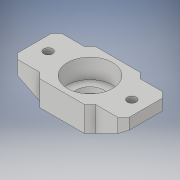
# Autodesk Inventor part: Sharrnir
Saved by Autodesk Inventor 2019.4 (Build 234330000, 330)
## iProperties
Created: 2019-04-09
Part Number: Sharrnir
Material: Типовые
Document SubType Name: Modeling
Designer: NoName
Density: 1 g/cm^3
Appearance: По умолчанию
Author: NoName
Autodesk Inventor part; units mm, degrees
ref_plane "YZ Plane" through (0, 0, 0) normal (1, 0, 0) x (0, 1, 0)
ref_plane "XZ Plane" through (0, 0, 0) normal (0, 1, 0) x (-1, 0, 0)
ref_plane "XY Plane" through (0, 0, 0) normal (0, 0, 1) x (1, 0, 0)
sketch "Эскиз1" plane through (0, 0, 0) normal (0, 1, 0) x (-1, 0, 0)
  circle A0 centre (0, 0) radius 5
  line L0 (8, 10) -> (-8, 10)
  line L1 (-10, 8) -> (-10, -8)
  line L2 (-8, -10) -> (8, -10)
  line L3 (10, -8) -> (10, 8)
  circle A1 centre (0, 0) radius 8 construction
  line L4 (8, 10) -> (10, 8)
  line L5 (10, -8) -> (8, -10)
  line L6 (-8, -10) -> (-10, -8)
  line L7 (-8, 10) -> (-10, 8)
  point P0 (10, 10)
  point P1 (-10, -10)
  point P2 (-10, 10)
  point P3 (10, -10)
  point P4 (0, -10)
  point P5 (10, 0)
  dimension "d0" = 10
  dimension "d3" = 16
  dimension "d4" = 20
  dimension "d5" = 20
  dimension "d6" = 2
  dimension "d7" = 2
  dimension "d8" = 2
  dimension "d9" = 2
  dimension "d10" = 2
  dimension "d11" = 2
  dimension "d12" = 2
  dimension "d13" = 2
  constraints: 16 end point, 8 point on line, 2 centre point, 2 coincident, 2 midpoint, 2 parallel, 1 horizontal, 1 horizontal alignment, 1 perpendicular, 1 vertical alignment
  measures "d0" diameter of A0
  measures "d3" diameter of A1
  measures "d4" distance between parallel lines of L2 L0
  measures "d5" distance between parallel lines of L3 L1
  measures "d6" distance of L0.start point (10, 10)
  measures "d7" distance of L3.end point (10, 10)
  measures "d8" distance of L3.start point (10, -10)
  measures "d9" distance of L2.end point (10, -10)
  measures "d10" distance of L2.start point (-10, -10)
  measures "d11" distance of L1.end point (-10, -10)
  measures "d12" distance of L0.end point (-10, 10)
  measures "d13" distance of L1.start point (-10, 10)
extrude "Выдавливание1" add sketch "Эскиз1" along normal blind 5
sketch "Эскиз4" plane through (0, 5, 0) normal (0, 1, 0) x (1, 0, 0)
  line L0 (12.8246, 0) -> (14.4123, 2.75) construction
  line L1 (14.4123, 2.75) -> (17.5877, 2.75) construction
  line L2 (17.5877, 2.75) -> (19.1754, 0) construction
  line L3 (19.1754, 0) -> (17.5877, -2.75) construction
  line L4 (17.5877, -2.75) -> (14.4123, -2.75) construction
  line L5 (14.4123, -2.75) -> (12.8246, 0) construction
  line L6 (10, -8) -> (20, -8)
  line L7 (20, -8) -> (20, 8)
  line L8 (20, 8) -> (10, 8)
  line L9 (8, -10) -> (10, -8) projected
  line L10 (10, -8) -> (8, -10)
  line L11 (8, -10) -> (0, -10)
  line L12 (8, -10) -> (-8, -10) projected
  line L13 (8, 10) -> (0, 10)
  line L14 (8, 10) -> (-8, 10) projected
  line L15 (10, 8) -> (8, 10) projected
  line L16 (10, 8) -> (8, 10)
  line L17 (0, -18.8546) -> (0, 18.8546)
  line L18 (-12.8246, 0) -> (-14.4123, 2.75) construction
  line L19 (-14.4123, 2.75) -> (-17.5877, 2.75) construction
  line L20 (-17.5877, 2.75) -> (-19.1754, 0) construction
  line L21 (-19.1754, 0) -> (-17.5877, -2.75) construction
  line L22 (-17.5877, -2.75) -> (-14.4123, -2.75) construction
  line L23 (-14.4123, -2.75) -> (-12.8246, 0) construction
  line L24 (-10, -8) -> (-20, -8)
  line L25 (-20, -8) -> (-20, 8)
  line L26 (-20, 8) -> (-10, 8)
  line L27 (-8, -10) -> (-10, -8)
  line L28 (-10, -8) -> (-8, -10)
  line L29 (-8, -10) -> (0, -10)
  line L30 (-8, 10) -> (0, 10)
  line L31 (-10, 8) -> (-8, 10)
  line L32 (-10, 8) -> (-8, 10)
  point P0 (0, 0)
  point P1 (16, 0)
  point P2 (0, 0)
  point P3 (-16, 0)
  dimension "d17" = 5.5
  dimension "d18" = 16
  dimension "d19" = 10
  constraints: 58 end point, 11 symmetric about line, 3 horizontal, 3 midpoint, 2 collinear, 1 coincident, 1 horizontal alignment, 1 perpendicular, 1 vertical, 13 other
  measures "d17" distance between parallel lines of L4 L1
  measures "d18" distance of point (0, 0) point (16, 0)
  measures "d19" distance of L6.start L6.end
extrude "Выдавливание2" add sketch "Эскиз4" along normal blind 4
sketch "Эскиз7" plane through (0, 9, 0) normal (0, 1, 0) x (1, 0, 0)
  circle A0 centre (0, 0) radius 8.1
  dimension "d26" = 16.2
  constraints: 1 centre point, 1 coincident
  measures "d26" diameter of A0
extrude "Выдавливание4" cut sketch "Эскиз7" against normal blind 7
sketch "Эскиз10" plane through (-10, 5, -8) normal (0, 0, -1) x (-1, 0, 0)
  line L0 (10, 0) -> (10, 4) projected
  line L1 (-2, -5) -> (0, -5) projected
  line L2 (10, 0) -> (0, -5)
  line L3 (0, -5) -> (0, 0)
  line L4 (10, 0) -> (0, 0) projected
  line L5 (0, 0) -> (10, 0)
  point P0 (-10, -5)
  constraints: 6 end point, 2 perpendicular
extrude "Выдавливание5" add sketch "Эскиз10" against normal blind 3
mirror "Зеркальное отражение1" about plane through (0, 0, 0) normal (0, 0, 1) of "Выдавливание5"
mirror "Зеркальное отражение2" about plane through (0, 0, 0) normal (1, 0, 0) of "Выдавливание5", "Зеркальное отражение1"
chamfer "Фаска1" distance 2 angle 45 4 edges at (-20, 7, -8) (20, 7, -8) (20, 7, 8) (-20, 7, 8)
sketch "Эскиз11" plane through (0, 5, 0) normal (0, -1, 0) x (1, 0, 0)
  point P0 (0, 0)
  point P1 (15, 0)
  point P2 (-15, 0)
  dimension "d48" = 30
  dimension "d49" = 15
  constraints: 2 horizontal alignment
  measures "d48" distance of point (15, 0) point (-15, 0)
  measures "d49" distance of point (-15, 0) point (0, 0)
hole "Отверстие2" at (15, 5, 0) at (-15, 5, 0) direction (0, 1, 0) diameter 3.2 end through all
equation "\"d7\" = d6"
equation "\"d8\" = d6"
equation "\"d9\" = d8"
equation "\"d10\" = d6"
equation "\"d11\" = d10"
equation "\"d12\" = d6"
equation "\"d13\" = d12"
